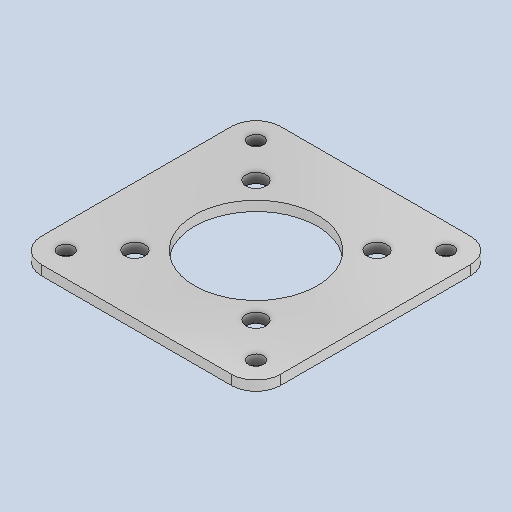
# Autodesk Inventor part: omu_al_jo_2
Saved by Autodesk Inventor 2025.1 (Build 291241000, 241)
## iProperties
Created: 2024-03-23
Part Number: omu_al_jo_2
Material: アルミニウム 6061-AHC
Document SubType Name: Modeling
Designer: fhbdh
Density: 2.7 g/cm^3
Appearance: アルミニウム - ダーク
Author: fhbdh
Autodesk Inventor part; units mm, degrees
ref_plane "YZ Plane" through (0, 0, 0) normal (1, 0, 0) x (0, 1, 0)
ref_plane "XZ Plane" through (0, 0, 0) normal (0, 1, 0) x (-1, 0, 0)
ref_plane "XY Plane" through (0, 0, 0) normal (0, 0, 1) x (1, 0, 0)
sketch "スケッチ1" plane through (0, 0, 0) normal (0, 1, 0) x (-1, 0, 0)
  circle A0 centre (0, 0) radius 12.55
  line L0 (0, 0) -> (0, -12.55) construction
  circle A1 centre (12.3744, -12.3744) radius 2.05
  line L1 (0, 0) -> (8.8742, -8.8742) construction
  circle A2 centre (19.4454, -19.4454) radius 1.55
  circle A3 centre (0, 0) radius 27.5 construction
  circle A4 centre (19.4454, 19.4454) radius 1.55
  circle A5 centre (-19.4454, 19.4454) radius 1.55
  circle A6 centre (-19.4454, -19.4454) radius 1.55
  line L2 (-24.4454, 24.4454) -> (24.4454, 24.4454)
  line L3 (24.4454, 24.4454) -> (24.4454, -24.4454)
  line L4 (24.4454, -24.4454) -> (-24.4454, -24.4454)
  line L5 (-24.4454, -24.4454) -> (-24.4454, 24.4454)
  line L6 (-24.4454, 24.4454) -> (24.4454, -24.4454) construction
  line L7 (24.4454, 24.4454) -> (-24.4454, -24.4454) construction
  circle A7 centre (12.3744, 12.3744) radius 2.05
  circle A8 centre (-12.3744, 12.3744) radius 2.05
  circle A9 centre (-12.3744, -12.3744) radius 2.05
  dimension "d9" = 55
  dimension "d0" = 25.1
  dimension "d1" = 4.1
  dimension "d7" = 45
  dimension "d8" = 3.1
  dimension "d12" = 360
  dimension "d14" = 5
  dimension "d20" = 360
  dimension "d22" = 35
  constraints: 16 end point, 9 centre point, 3 point on line, 2 coincident, 2 midpoint, 2 parallel, 2 point on circle, 1 horizontal, 1 perpendicular, 1 vertical, 21 other
  measures "d0" diameter of A0
  measures "d1" diameter of A1
  measures "d7" angle of L0 L1
  measures "d8" diameter of A2
  measures "d14" distance from line of L4 A2.centre
  measures "d22" distance of A8.centre A1.centre
extrude "押し出し1" add sketch "スケッチ1" along normal blind 2
fillet "フィレット1" radius 5 4 edges at (24.4454, 1, 24.4454) (24.4454, 1, -24.4454) (-24.4454, 1, -24.4454) (-24.4454, 1, 24.4454)
sketch "スケッチ2" plane through (0, 2, 0) normal (0, 1, 0) x (1, 0, 0)
  arc A0 (-24.4454, -19.4454) -> (-19.4454, -24.4454) centre (-19.4454, -19.4454) ccw projected
  line L0 (-19.4454, -24.4454) -> (19.4454, -24.4454) projected
  arc A1 (19.4454, -24.4454) -> (24.4454, -19.4454) centre (19.4454, -19.4454) ccw projected
  line L1 (24.4454, -19.4454) -> (24.4454, 19.4454) projected
  arc A2 (24.4454, 19.4454) -> (19.4454, 24.4454) centre (19.4454, 19.4454) ccw projected
  line L2 (19.4454, 24.4454) -> (-19.4454, 24.4454) projected
  arc A3 (-19.4454, 24.4454) -> (-24.4454, 19.4454) centre (-19.4454, 19.4454) ccw projected
  line L3 (-24.4454, 19.4454) -> (-24.4454, -19.4454) projected
  circle A4 centre (-19.4454, 19.4454) radius 1.55 projected
  circle A5 centre (-19.4454, -19.4454) radius 1.55 projected
  circle A6 centre (19.4454, -19.4454) radius 1.55 projected
  circle A7 centre (19.4454, 19.4454) radius 1.55 projected
  circle A8 centre (12.3744, 12.3744) radius 2.05 projected
  circle A9 centre (12.3744, -12.3744) radius 2.05 projected
  circle A10 centre (-12.3744, -12.3744) radius 2.05 projected
  circle A11 centre (-12.3744, 12.3744) radius 2.05 projected
  circle A12 centre (0, 0) radius 12.55 projected
